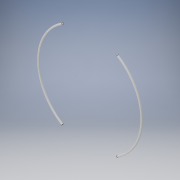
# Autodesk Inventor part: PossibleTopCapBallHolder
Saved by Autodesk Inventor 2017 (Build 210142000, 142)
## iProperties
Created: 2017-06-14
Part Number: PossibleTopCapBallHolder
Material: Generic
Document SubType Name: Modeling
Designer: User
Density: 1 g/cm^3
Appearance: Default
Author: User
Autodesk Inventor part; units mm, degrees
ref_plane "YZ Plane" through (0, 0, 0) normal (1, 0, 0) x (0, 1, 0)
ref_plane "XZ Plane" through (0, 0, 0) normal (0, 1, 0) x (-1, 0, 0)
ref_plane "XY Plane" through (0, 0, 0) normal (0, 0, 1) x (1, 0, 0)
sketch "Sketch1" plane through (0, 0, 0) normal (0, 0, 1) x (1, 0, 0)
  arc A0 (-101.6, 161.1449) -> (-101.6, -161.1449) centre (0, 0) ccw
  arc A1 (101.6, -161.1449) -> (101.6, 161.1449) centre (0, 0) ccw
  point P0 (0, 0)
  constraints: 4 point on circle, 2 centre point
ref_plane "Work Plane5" through (101.6, 161.1449, 0) normal (-0.8459052, 0.5333333, 0) x (-0.5333333, -0.8459052, 0)
ref_plane "Work Plane6" through (-101.6, 161.1449, 0) normal (-0.8459052, -0.5333333, 0) x (0.5333333, -0.8459052, 0)
sketch "Sketch4" plane through (-101.6, 161.1449, 0) normal (-0.8459052, -0.5333333, 0) x (0.5333333, -0.8459052, 0)
  circle A0 centre (0, 0) radius 3.175
  point P0 (190.5, 0)
  dimension "d3" = 6.35
  constraints: 1 centre point
  measures "d3" diameter of A0
sketch "Sketch5" plane through (101.6, 161.1449, 0) normal (-0.8459052, 0.5333333, 0) x (-0.5333333, -0.8459052, 0)
  circle A0 centre (0, 0) radius 3.175
  point P0 (190.5, 0)
  dimension "d4" = 6.35
  constraints: 1 centre point
  measures "d4" diameter of A0
sweep "Sweep1" add profiles "Sketch4" path "Sketch1" path curves A0
sweep "Sweep2" add profiles "Sketch5" path "Sketch1" path curves A1
body "Solid1"
